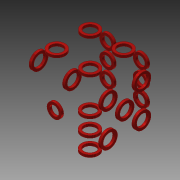
# Autodesk Inventor part: Dice
Saved by Autodesk Inventor 2013 (Build 170138000, 138)
## iProperties
Created: 2013-02-11
Part Number: Dice
Material: Generic
Document SubType Name: Modeling
Designer: rhys
Density: 1 g/cm^3
Author: rhys
Autodesk Inventor part; units mm, degrees
ref_plane "YZ Plane" through (0, 0, 0) normal (1, 0, 0) x (0, 1, 0)
ref_plane "XZ Plane" through (0, 0, 0) normal (0, 1, 0) x (-1, 0, 0)
sketch "Sketch1" plane through (0, 0, 0) normal (0, 1, 0) x (-1, 0, 0)
  line L0 (15, -15) -> (-15, -15)
  line L1 (-15, -15) -> (-15, 15)
  line L2 (-15, 15) -> (15, 15)
  line L3 (15, 15) -> (15, -15)
  line L4 (15, -15) -> (-15, 15) construction
  line L5 (-15, -15) -> (15, 15) construction
  point P0 (0, 0)
  dimension "d0" = 30
  dimension "d2" = 30
  constraints: 12 end point, 2 midpoint, 2 parallel, 1 horizontal, 1 perpendicular
  measures "d0" distance of L1.end L2.end
  measures "d2" distance of L2.end L0.start
extrude "Extrusion1" add sketch "Sketch1" along normal blind 30
fillet "Fillet1" radius 4 12 edges at (0, 0, 15) (15, 15, 15) (0, 30, 15) (-15, 15, 15) (15, 0, 0) (15, 15, -15) (15, 30, 0) (0, 30, -15) (-15, 30, 0) (0, 0, -15) (-15, 15, -15) (-15, 0, 0)
sketch "Sketch2" plane through (0, 0, 0) normal (0, -1, 0) x (1, 0, 0)
  circle A0 centre (0, 0) radius 3
  dimension "d6" = 6
  constraints: 1 centre point
  measures "d6" diameter of A0
extrude "Extrusion2" cut sketch "Sketch2" against normal blind 1
sketch "Sketch3" plane through (0, 30, 0) normal (0, 1, 0) x (1, 0, 0)
  circle A0 centre (-7, 0) radius 3
  circle A1 centre (-7, 7) radius 3
  circle A2 centre (-7, -7) radius 3
  point P0 (0, 0)
  dimension "d11" = 6
  dimension "d13" = 6
  dimension "d14" = 6
  dimension "d15" = 7
  dimension "d16" = 7
  dimension "d17" = 0
  dimension "d18" = 7
  dimension "d19" = 0
  constraints: 3 centre point
  measures "d11" diameter of A0
  measures "d13" diameter of A1
  measures "d14" diameter of A2
  measures "d15" distance of A0.centre A1.centre
  measures "d16" distance of A2.centre A0.centre
  measures "d17" vertical distance of A0.centre point (0, 0)
  measures "d18" horizontal distance of point (0, 0) A1.centre
  measures "d19" horizontal distance of A0.centre A1.centre
extrude "Extrusion3" cut sketch "Sketch3" against normal blind 1
ref_plane "Work Plane1" through (0, 4, 11) normal (-1, 0, 0) x (0, 0, 1)
mirror "Mirror1" about plane through (0, 4, 11) normal (-1, 0, 0) of "Extrusion3"
sketch "Sketch4" plane through (-11, 26, 15) normal (0, 0, 1) x (1, 0, 0)
  line L0 (17.9652, -17.8811) -> (3.9652, -17.8811) construction
  line L1 (3.9652, -17.8811) -> (3.9652, -3.8811) construction
  line L2 (3.9652, -3.8811) -> (17.9652, -3.8811) construction
  line L3 (17.9652, -3.8811) -> (17.9652, -17.8811) construction
  line L4 (17.9652, -17.8811) -> (3.9652, -3.8811) construction
  line L5 (3.9652, -17.8811) -> (17.9652, -3.8811) construction
  circle A0 centre (3.9652, -3.8811) radius 3.5
  circle A1 centre (3.9652, -17.8811) radius 3.5
  circle A2 centre (17.9652, -17.8811) radius 3.5
  circle A3 centre (17.9652, -3.8811) radius 3.5
  point P0 (11, -26)
  point P1 (10.9652, -10.8811)
  dimension "d22" = 7
  dimension "d23" = 7
  dimension "d24" = 7
  dimension "d25" = 7
  dimension "d28" = 14
  dimension "d29" = 14
  constraints: 12 end point, 4 centre point, 4 coincident, 2 midpoint, 2 parallel, 1 horizontal, 1 perpendicular
  measures "d22" diameter of A0
  measures "d23" diameter of A1
  measures "d24" diameter of A2
  measures "d25" diameter of A3
  measures "d28" distance of L1.end L2.end
  measures "d29" distance of L2.end L0.start
extrude "Extrusion4" cut sketch "Sketch4" against normal blind 1
sketch "Sketch5" plane through (11, 4, -15) normal (0, 0, -1) x (-1, 0, 0)
  line L0 (0, 22) -> (22, 22) projected
  line L1 (0, 0) -> (0, 22) projected
  line L2 (18, 4) -> (4, 4)
  line L3 (4, 4) -> (4, 18)
  line L4 (4, 18) -> (18, 18)
  line L5 (18, 18) -> (18, 4)
  line L6 (18, 4) -> (4, 18) construction
  line L7 (4, 4) -> (18, 18) construction
  circle A0 centre (18, 18) radius 3.5
  circle A1 centre (4, 4) radius 3.5
  circle A2 centre (11, 11) radius 3.5
  point P0 (11, -4)
  dimension "d30" = 14
  dimension "d32" = 14
  dimension "d33" = 4
  dimension "d34" = 4
  dimension "d35" = 7
  dimension "d36" = 7
  dimension "d39" = 7
  constraints: 12 end point, 3 centre point, 3 coincident, 2 midpoint, 2 parallel, 1 horizontal, 1 perpendicular
  measures "d30" distance of L3.end L4.end
  measures "d32" distance of L2.end L3.end
  measures "d33" distance between parallel lines of L1 L3
  measures "d34" distance between parallel lines of L0 L4
  measures "d35" diameter of A1
  measures "d36" diameter of A0
  measures "d39" diameter of A2
extrude "Extrusion5" cut sketch "Sketch5" against normal blind 1 contours A1 L3 L2 | L2 L3 A1 | A0 L4 L5 | L5 L4 A0 | A2
sketch "Sketch6" plane through (-15, 4, 11) normal (-1, 0, 0) x (0, 0, 1)
  line L0 (0, 22) -> (0, 0) projected
  line L1 (-22, 22) -> (0, 22) projected
  line L2 (-4, 4) -> (-18, 4)
  line L3 (-18, 4) -> (-18, 18)
  line L4 (-18, 18) -> (-4, 18)
  line L5 (-4, 18) -> (-4, 4)
  line L6 (-4, 4) -> (-18, 18) construction
  line L7 (-18, 4) -> (-4, 18) construction
  circle A0 centre (-18, 18) radius 3.5
  circle A1 centre (-4, 4) radius 3.5
  point P0 (-11, -4)
  point P1 (-11, 11)
  dimension "d40" = 14
  dimension "d42" = 14
  dimension "d43" = 4
  dimension "d44" = 4
  dimension "d45" = 7
  dimension "d46" = 7
  constraints: 12 end point, 2 centre point, 2 coincident, 2 midpoint, 2 parallel, 1 horizontal, 1 perpendicular
  measures "d40" distance of L3.end L4.end
  measures "d42" distance of L2.end L3.end
  measures "d43" distance between parallel lines of L1 L4
  measures "d44" distance between parallel lines of L0 L5
  measures "d45" diameter of A0
  measures "d46" diameter of A1
extrude "Extrusion6" cut sketch "Sketch6" against normal blind 1 contours L5 A1 L2 | L2 A1 L5 | A0 L4 L3 | L3 L4 A0
sketch "Sketch7" plane through (15, 4, -11) normal (1, 0, 0) x (0, 0, -1)
  line L0 (-22, 22) -> (0, 22) projected
  line L1 (-22, 0) -> (-22, 22) projected
  line L2 (-4, 4) -> (-18, 4)
  line L3 (-18, 4) -> (-18, 18)
  line L4 (-18, 18) -> (-4, 18)
  line L5 (-4, 18) -> (-4, 4)
  line L6 (-4, 4) -> (-18, 18) construction
  line L7 (-18, 4) -> (-4, 18) construction
  circle A0 centre (-18, 18) radius 3.5
  circle A1 centre (-18, 4) radius 3.5
  circle A2 centre (-4, 4) radius 3.5
  circle A3 centre (-4, 18) radius 3.5
  circle A4 centre (-11, 11) radius 3.5
  point P0 (-11, -4)
  dimension "d49" = 14
  dimension "d51" = 14
  dimension "d52" = 4
  dimension "d53" = 4
  dimension "d54" = 7
  dimension "d55" = 7
  dimension "d56" = 7
  dimension "d57" = 7
  dimension "d58" = 7
  constraints: 12 end point, 5 centre point, 5 coincident, 2 midpoint, 2 parallel, 1 horizontal, 1 perpendicular
  measures "d49" distance of L3.end L4.end
  measures "d51" distance of L2.end L3.end
  measures "d52" distance between parallel lines of L1 L3
  measures "d53" distance between parallel lines of L0 L4
  measures "d54" diameter of A0
  measures "d55" diameter of A3
  measures "d56" diameter of A4
  measures "d57" diameter of A1
  measures "d58" diameter of A2
extrude "Extrusion7" cut sketch "Sketch7" against normal blind 1 contours A1 L3 L2 | L2 L3 A1 | A2 L5 L2 | L2 L5 A2 | A0 L4 L3 | L3 L4 A0 | A3 L4 L5 | L5 L4 A3 | A4
sketch "Sketch8" plane through (11, 4, -15) normal (0, 0, -1) x (-1, 0, 0)
  circle A0 centre (11, 11) radius 3.5 projected
  circle A1 centre (18, 18) radius 3.5 projected
  circle A2 centre (4, 4) radius 3.5 projected
  circle A3 centre (18, 18) radius 2.5
  circle A4 centre (11, 11) radius 2.5
  circle A5 centre (4, 4) radius 2.5
  point P0 (11, -4)
  dimension "d63" = 1
  dimension "d64" = 1
  dimension "d65" = 1
  constraints: 3 centre point
  measures "d63" radial gap between concentric circles of A2 A5
  measures "d64" radial gap between concentric circles of A0 A4
  measures "d65" radial gap between concentric circles of A1 A3
sketch "Sketch9" plane through (15, 4, -11) normal (1, 0, 0) x (0, 0, -1)
  circle A0 centre (-11, 11) radius 3.5 projected
  circle A1 centre (-4, 4) radius 3.5 projected
  circle A2 centre (-18, 18) radius 3.5 projected
  circle A3 centre (-18, 4) radius 3.5 projected
  circle A4 centre (-4, 18) radius 3.5 projected
  circle A5 centre (-18, 18) radius 2.5
  circle A6 centre (-4, 18) radius 2.5
  circle A7 centre (-11, 11) radius 2.5
  circle A8 centre (-4, 4) radius 2.5
  circle A9 centre (-18, 4) radius 2.5
  point P0 (-11, -4)
  dimension "d66" = 1
  dimension "d67" = 1
  dimension "d68" = 1
  dimension "d69" = 1
  dimension "d70" = 1
  constraints: 5 centre point
  measures "d66" radial gap between concentric circles of A2 A5
  measures "d67" radial gap between concentric circles of A4 A6
  measures "d68" radial gap between concentric circles of A0 A7
  measures "d69" radial gap between concentric circles of A3 A9
  measures "d70" radial gap between concentric circles of A1 A8
sketch "Sketch10" plane through (-11, 26, 15) normal (0, 0, 1) x (1, 0, 0)
  circle A0 centre (17.9652, -17.8811) radius 3.5 projected
  circle A1 centre (3.9652, -3.8811) radius 3.5 projected
  circle A2 centre (3.9652, -17.8811) radius 3.5 projected
  circle A3 centre (17.9652, -3.8811) radius 3.5 projected
  circle A4 centre (3.9652, -3.8811) radius 2.5
  circle A5 centre (17.9652, -3.8811) radius 2.5
  circle A6 centre (17.9652, -17.8811) radius 2.5
  circle A7 centre (3.9652, -17.8811) radius 2.5
  point P0 (11, -26)
  dimension "d71" = 1
  dimension "d72" = 1
  dimension "d73" = 1
  dimension "d74" = 1
  constraints: 4 centre point
  measures "d71" radial gap between concentric circles of A1 A4
  measures "d72" radial gap between concentric circles of A3 A5
  measures "d73" radial gap between concentric circles of A6 A0
  measures "d74" radial gap between concentric circles of A7 A2
sketch "Sketch11" plane through (-15, 4, 11) normal (-1, 0, 0) x (0, 0, 1)
  circle A0 centre (-4, 4) radius 3.5 projected
  circle A1 centre (-18, 18) radius 3.5 projected
  circle A2 centre (-18, 18) radius 2.5
  circle A3 centre (-4, 4) radius 2.5
  point P0 (-11, -4)
  dimension "d75" = 1
  dimension "d76" = 5
  constraints: 2 centre point
  measures "d75" radial gap between concentric circles of A1 A2
  measures "d76" diameter of A3
sketch "Sketch12" plane through (0, 30, 0) normal (0, 1, 0) x (1, 0, 0)
  circle A0 centre (7, 7) radius 3 projected
  circle A1 centre (7, 0) radius 3 projected
  circle A2 centre (7, -7) radius 3 projected
  circle A3 centre (-7, 7) radius 3 projected
  circle A4 centre (-7, 0) radius 3 projected
  circle A5 centre (-7, -7) radius 3 projected
  circle A6 centre (-7, 0) radius 2
  circle A7 centre (-7, 7) radius 2
  circle A8 centre (7, 7) radius 2
  circle A9 centre (7, 0) radius 2
  circle A10 centre (7, -7) radius 2
  circle A11 centre (-7, -7) radius 2
  point P0 (0, 0)
  dimension "d77" = 1
  dimension "d78" = 1
  dimension "d79" = 1
  dimension "d80" = 1
  dimension "d81" = 1
  dimension "d82" = 1
  constraints: 6 centre point
  measures "d77" radial gap between concentric circles of A3 A7
  measures "d78" radial gap between concentric circles of A6 A4
  measures "d79" radial gap between concentric circles of A5 A11
  measures "d80" radial gap between concentric circles of A10 A2
  measures "d81" radial gap between concentric circles of A9 A1
  measures "d82" radial gap between concentric circles of A8 A0
sketch "Sketch13" plane through (0, 0, 0) normal (0, -1, 0) x (1, 0, 0)
  circle A0 centre (0, 0) radius 3 projected
  circle A1 centre (0, 0) radius 2
  dimension "d85" = 1
  constraints: 1 centre point
  measures "d85" radial gap between concentric circles of A0 A1
sketch "Sketch15" plane through (-15, 4, 11) normal (-1, 0, 0) x (0, 0, 1)
  line L0 (11.0554, -8.3661) -> (-31.3706, -8.3661)
  line L1 (-31.3706, -8.3661) -> (-31.3706, 30.3661)
  line L2 (-31.3706, 30.3661) -> (11.0554, 30.3661)
  line L3 (11.0554, 30.3661) -> (11.0554, -8.3661)
  line L4 (11.0554, -8.3661) -> (-31.3706, 30.3661) construction
  line L5 (-31.3706, -8.3661) -> (11.0554, 30.3661) construction
  point P0 (-11, -4)
  point P1 (-10.1576, 11)
  constraints: 12 end point, 2 midpoint, 2 parallel, 1 horizontal, 1 perpendicular
extrude "Extrusion8" cut sketch "Sketch15" along normal through all both and the other way through all
extrude "Extrusion9" add sketch "Sketch13" against normal blind 1 contours A1
extrude "Extrusion10" add sketch "Sketch11" against normal blind 1 contours A2 | A3
extrude "Extrusion11" add sketch "Sketch10" against normal blind 1 contours A4 | A5 | A6 | A7
extrude "Extrusion12" add sketch "Sketch12" against normal blind 1 contours A6 | A7 | A8 | A9 | A10 | A11
extrude "Extrusion13" add sketch "Sketch8" against normal blind 1 contours A3 | A4 | A5
extrude "Extrusion14" add sketch "Sketch9" against normal blind 1 contours A5 | A6 | A7 | A8 | A9
sketch "Sketch16" plane through (0, 30, 0) normal (0, 1, 0) x (1, 0, 0)
  circle A0 centre (7, 7) radius 3 projected
  circle A1 centre (7, 0) radius 3 projected
  circle A2 centre (7, -7) radius 3 projected
  circle A3 centre (-7, 7) radius 3 projected
  circle A4 centre (-7, 0) radius 3 projected
  circle A5 centre (-7, -7) radius 3 projected
  circle A6 centre (-7, 7) radius 2 projected
  circle A7 centre (7, 7) radius 2 projected
  circle A8 centre (7, 0) radius 2 projected
  circle A9 centre (-7, 0) radius 2 projected
  circle A10 centre (-7, -7) radius 2 projected
  circle A11 centre (7, -7) radius 2 projected
  point P0 (0, 0)
sketch "Sketch17" plane through (11, 4, -15) normal (0, 0, -1) x (-1, 0, 0)
  circle A0 centre (11, 11) radius 3.5 projected
  circle A1 centre (18, 18) radius 3.5 projected
  circle A2 centre (4, 4) radius 3.5 projected
  circle A3 centre (11, 11) radius 2.5 projected
  circle A4 centre (18, 18) radius 2.5 projected
  circle A5 centre (4, 4) radius 2.5 projected
  point P0 (11, -4)
sketch "Sketch18" plane through (15, 4, -11) normal (1, 0, 0) x (0, 0, -1)
  circle A0 centre (-11, 11) radius 3.5 projected
  circle A1 centre (-4, 4) radius 3.5 projected
  circle A2 centre (-18, 18) radius 3.5 projected
  circle A3 centre (-18, 4) radius 3.5 projected
  circle A4 centre (-4, 18) radius 3.5 projected
  circle A5 centre (-18, 18) radius 2.5 projected
  circle A6 centre (-4, 18) radius 2.5 projected
  circle A7 centre (-11, 11) radius 2.5 projected
  circle A8 centre (-18, 4) radius 2.5 projected
  circle A9 centre (-4, 4) radius 2.5 projected
  point P0 (-11, -4)
sketch "Sketch19" plane through (-11, 26, 15) normal (0, 0, 1) x (1, 0, 0)
  circle A0 centre (17.9652, -17.8811) radius 3.5 projected
  circle A1 centre (3.9652, -3.8811) radius 3.5 projected
  circle A2 centre (3.9652, -17.8811) radius 3.5 projected
  circle A3 centre (17.9652, -3.8811) radius 3.5 projected
  circle A4 centre (3.9652, -3.8811) radius 2.5 projected
  circle A5 centre (17.9652, -3.8811) radius 2.5 projected
  circle A6 centre (17.9652, -17.8811) radius 2.5 projected
  circle A7 centre (3.9652, -17.8811) radius 2.5 projected
  point P0 (11, -26)
sketch "Sketch20" plane through (-15, 4, 11) normal (-1, 0, 0) x (0, 0, 1)
  circle A0 centre (-4, 4) radius 3.5 projected
  circle A1 centre (-18, 18) radius 3.5 projected
  circle A2 centre (-18, 18) radius 2.5 projected
  circle A3 centre (-4, 4) radius 2.5 projected
  point P0 (-11, -4)
sketch "Sketch21" plane through (0, 0, 0) normal (0, -1, 0) x (1, 0, 0)
  circle A0 centre (0, 0) radius 3 projected
  circle A1 centre (0, 0) radius 2 projected
sketch "Sketch23" plane through (0, 15, -14) normal (0, 0, 1) x (1, 0, 0)
  circle A0 centre (0, 0) radius 2.5 projected
  line L0 (18.9155, -17.8731) -> (-18.9155, -17.8731)
  line L1 (-18.9155, -17.8731) -> (-18.9155, 17.8731)
  line L2 (-18.9155, 17.8731) -> (18.9155, 17.8731)
  line L3 (18.9155, 17.8731) -> (18.9155, -17.8731)
  line L4 (18.9155, -17.8731) -> (-18.9155, 17.8731) construction
  line L5 (-18.9155, -17.8731) -> (18.9155, 17.8731) construction
  point P0 (0, -15)
  constraints: 12 end point, 2 midpoint, 2 parallel, 1 horizontal, 1 perpendicular
extrude "Extrusion16" cut sketch "Sketch23" along normal mid plane 100 contours A0 | L0 L1 L2 L3
extrude "Extrusion17" add sketch "Sketch16" against normal blind 1
extrude "Extrusion18" add sketch "Sketch19" against normal blind 1
extrude "Extrusion19" add sketch "Sketch20" against normal blind 1
extrude "Extrusion20" add sketch "Sketch17" against normal blind 1
extrude "Extrusion21" add sketch "Sketch18" against normal blind 1
extrude "Extrusion22" add sketch "Sketch21" against normal blind 1
body "Solid1"
